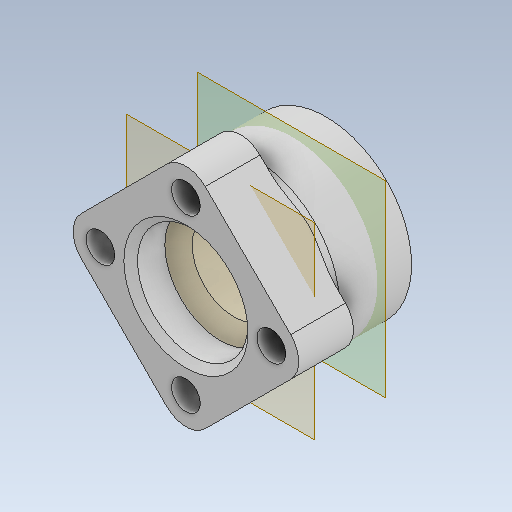
# Autodesk Inventor part: bearing_shell_1
Saved by Autodesk Inventor 2020 (Build 240168000, 168)
## iProperties
Created: 2020-07-16
Part Number: bearing_shell_1
Material: Generic
Document SubType Name: Modeling
Designer: psrobotics
Density: 1 g/cm^3
Appearance: Default
Author: psrobotics
Autodesk Inventor part; units mm, degrees
ref_plane "YZ Plane" through (0, 0, 0) normal (1, 0, 0) x (0, 1, 0)
ref_plane "XZ Plane" through (0, 0, 0) normal (0, 1, 0) x (-1, 0, 0)
sketch "Sketch1" plane through (0, 0, 0) normal (0, 0, 1) x (1, 0, 0)
  circle A0 centre (0, 0) radius 5.075 projected
  circle A1 centre (0, 0) radius 8.075
  circle A2 centre (0, 0) radius 12.5
  point P0 (0, 0)
  dimension "d0" = 16.15
  dimension "d1" = 25
  constraints: 2 centre point, 2 coincident
  measures "d0" diameter of A1
  measures "d1" diameter of A2
ref_plane "Work Plane1" through (-35.929292, -119.395492, 20.5) normal (0, 0, -1) x (-0.2157999, 0.9764376, 0)
extrude "Extrusion1" add sketch "Sketch1" along normal up to surface (20.5 mm away) contours A2
ref_plane "Work Plane2" through (0, 0, 15.5) normal (0, 0, 1) x (1, 0, 0)
ref_plane "Work Plane3" through (0, 0, 5) normal (0, 0, -1) x (-1, 0, 0)
sketch "Sketch2" plane through (0, 0, 5) normal (0, 0, -1) x (-1, 0, 0)
  circle A0 centre (0, 0) radius 8.075 projected
  circle A1 centre (0, 0) radius 6.075
  point P0 (0, 0)
  dimension "d6" = 2
  constraints: 1 centre point, 1 coincident
  measures "d6" radial gap between concentric circles of A0 A1
extrude "Extrusion2" add sketch "Sketch2" against normal up to surface (10.5 mm away)
chamfer "Chamfer1" distance 2 angle 45 2 edges at (6.075, 0, 5) (6.075, 0, 15.5)
sketch "Sketch3" plane through (0, 0, 20.5) normal (0, 0, 1) x (1, 0, 0)
  circle A0 centre (0, 0) radius 8.075 projected
  circle A1 centre (0, 0) radius 12.5 projected
  line L0 (0, 0) -> (12.5, 0)
  circle A2 centre (0, 0) radius 12.5 projected
  circle A3 centre (12.5, 0) radius 4
  point P0 (0, 0)
  dimension "d12" = 8
  constraints: 2 end point, 1 centre point, 1 coincident, 1 horizontal, 1 horizontal alignment, 1 other
  measures "d12" diameter of A3
extrude "Extrusion3" add sketch "Sketch3" against normal blind 8 contours L0 A3 A1 | A1 A3 | A1 A3 L0 picked at (13.649589, -1.078546)
pattern_circular "Circular Pattern1" count 4 over 360 about axis through (0, 0, 0) along (0, 0, 1) of "Extrusion3"
sketch "Sketch6" plane through (12.5, 0, 20.5) normal (0, 0, 1) x (1, 0, 0)
  arc A0 (-8.551532, -11.86) -> (-0.64, -3.948468) centre (-12.5, 0) ccw
  arc A1 (-0.64, -3.948468) -> (-0.64, 3.948468) centre (0, 0) ccw
  arc A2 (-0.64, 3.948468) -> (-8.551532, 11.86) centre (-12.5, 0) ccw
  arc A3 (-8.551532, 11.86) -> (-16.448468, 11.86) centre (-12.5, 12.5) ccw
  arc A4 (-16.448468, 11.86) -> (-24.36, 3.948468) centre (-12.5, 0) ccw
  arc A5 (-24.36, 3.948468) -> (-24.36, -3.948468) centre (-25, 0) ccw
  arc A6 (-24.36, -3.948468) -> (-16.448468, -11.86) centre (-12.5, 0) ccw
  arc A7 (-16.448468, -11.86) -> (-8.551532, -11.86) centre (-12.5, -12.5) ccw
  circle A8 centre (-12.5, 0) radius 8.075
  line L0 (-12.5, 12.5) -> (-15.328427, 15.328427)
  arc A9 (-8.551532, 11.86) -> (-16.448468, 11.86) centre (-12.5, 12.5) ccw
  line L1 (-25, 0) -> (-27.828427, 2.828427)
  line L2 (-27.828427, 2.828427) -> (-15.328427, 15.328427)
  point P0 (-12.5, 0)
  constraints: 6 end point, 2 perpendicular, 2 point on circle
extrude "Extrusion5" add sketch "Sketch6" against normal blind 8 contours L2 A3 A4 A5
pattern_circular "Circular Pattern3" count 4 over 360 about axis through (0, 0, 0) along (0, 0, 1) of "Extrusion5"
sketch "Sketch7" plane through (0, 12.5, 20.5) normal (0, 0, 1) x (1, 0, 0)
  arc A0 (15.328427, -15.328427) -> (15.328427, -9.671573) centre (12.5, -12.5) ccw
  line L0 (15.328427, -9.671573) -> (2.828427, 2.828427)
  arc A1 (2.828427, 2.828427) -> (-2.828427, 2.828427) centre (0, 0) ccw
  line L1 (-2.828427, 2.828427) -> (-15.328427, -9.671573)
  arc A2 (-15.328427, -9.671573) -> (-15.328427, -15.328427) centre (-12.5, -12.5) ccw
  line L2 (-15.328427, -15.328427) -> (-2.828427, -27.828427)
  arc A3 (-2.828427, -27.828427) -> (2.828427, -27.828427) centre (0, -25) ccw
  line L3 (2.828427, -27.828427) -> (15.328427, -15.328427)
  circle A4 centre (0, -12.5) radius 8.075
  circle A5 centre (-12.5, -12.5) radius 2.1
  point P0 (0, -12.5)
  dimension "d29" = 4.2
  constraints: 1 centre point, 1 coincident
  measures "d29" diameter of A5
extrude "Extrusion6" cut sketch "Sketch7" against normal blind 6 contours A5
pattern_circular "Circular Pattern4" count 4 over 360 about axis through (0, 0, 0) along (0, 0, 1) of "Extrusion6"
fillet "Fillet1" radius 2 1 edges at (-12.5, 0, 12.5)
chamfer "Chamfer2" distance 1 angle 45 2 edges at (-8.075, 0, 0) (-8.075, 0, 20.5)
body "Solid1"
